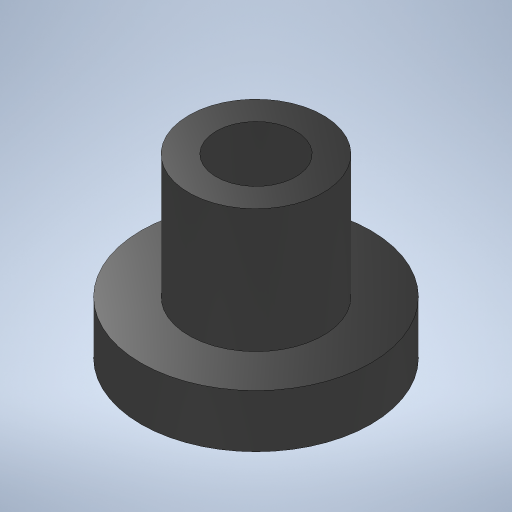
# Autodesk Inventor part: omu_3d_jo_5
Saved by Autodesk Inventor 2024.2 (Build 282272000, 272)
## iProperties
Created: 2024-03-24
Part Number: omu_3d_jo_5
Material: ABS プラスチック
Document SubType Name: Modeling
Designer: fhbdh
Density: 1.06 g/cm^3
Appearance: 光沢 - 黒
Author: fhbdh
Autodesk Inventor part; units mm, degrees
ref_plane "YZ Plane" through (0, 0, 0) normal (1, 0, 0) x (0, 1, 0)
ref_plane "XZ Plane" through (0, 0, 0) normal (0, 1, 0) x (-1, 0, 0)
ref_plane "XY Plane" through (0, 0, 0) normal (0, 0, 1) x (1, 0, 0)
sketch "スケッチ1" plane through (0, 0, 0) normal (0, 0, 1) x (1, 0, 0)
  line L0 (-2.25, 10) -> (-2.25, 0)
  line L1 (-2.25, 0) -> (-6.5, 0)
  line L2 (-6.5, 0) -> (-6.5, 3)
  line L3 (-6.5, 3) -> (-3.8, 3)
  line L4 (-3.8, 3) -> (-3.8, 10)
  line L5 (-3.8, 10) -> (-2.25, 10)
  line L6 (0, 0) -> (0, 10) construction
  dimension "d0" = 2.25
  dimension "d1" = 3.8
  dimension "d2" = 6.5
  dimension "d3" = 3
  dimension "d6" = 7
  constraints: 14 end point, 4 perpendicular, 2 point on line, 2 vertical, 1 horizontal
  measures "d0" distance from line of L6.start L0
  measures "d1" distance from line of L6.start L4
  measures "d2" distance from line of L6.start L2
  measures "d3" distance of L1.end L2.end
  measures "d6" distance of L3.end L4.end
revolve "回転1" add sketch "スケッチ1" angle 360 about axis through (0, 0, 0) along (0, 1, 0)
